Autodesk Inventor part; units mm, degrees
(part 2 of 2)
  measures "d192" distance of L198.end L196.start
extrude "Выдавливание10" cut sketch "Эскиз16" against normal blind 10
